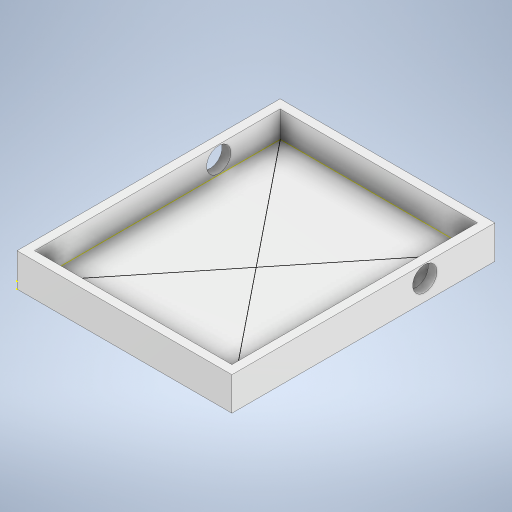
# Autodesk Inventor part: Case_3d_model2
Saved by Autodesk Inventor 2023 (Build 270158000, 158)
## iProperties
Created: 2023-03-21
Part Number: Case_3d_model2
Material: ABS Plastic
Document SubType Name: Sheet Metal
Designer: Inteli
Density: 1.06 g/cm^3
Sheet Metal Rule: Default
Appearance: Smooth - White
Author: Inteli
## iProperties of the stored document Case_3d_model_3DPrint.ipt
Created: 2023-03-23
Part Number: Case_3d_model_3DPrint
Material: Generic
Document SubType Name: Modeling
Designer: Inteli
Density: 1 g/cm^3
Appearance: Default
Author: Inteli
Autodesk Inventor part; units mm, degrees
ref_plane "YZ Plane" through (0, 0, 0) normal (1, 0, 0) x (0, 1, 0)
ref_plane "XZ Plane" through (0, 0, 0) normal (0, 1, 0) x (-1, 0, 0)
ref_plane "XY Plane" through (0, 0, 0) normal (0, 0, 1) x (1, 0, 0)
sketch "Sketch1" plane through (0, 0, 0) normal (0, 1, 0) x (-1, 0, 0)
  line L0 (0, 0) -> (0, -250)
  line L1 (-200, 0) -> (0, 0)
  line L2 (0, -250) -> (0, -300)
  line L3 (0, -300) -> (-200, -300)
  line L4 (-200, -300) -> (-230, -300)
  line L5 (-230, 0) -> (-200, 0)
  line L6 (-230, -300) -> (-245, -300)
  line L7 (-245, -300) -> (-245, 0)
  line L8 (-245, 0) -> (-230, 0)
  dimension "d0" = 250
  dimension "d4" = 50
  dimension "d12" = 30
  dimension "d24" = 15
  constraints: 18 end point, 2 horizontal, 2 perpendicular, 2 vertical
  measures "d0" distance of L0.start L0.end
  measures "d4" distance of L0.end L2.end
  measures "d12" distance of L3.end L4.end
  measures "d24" distance of L4.end L6.end
extrude "Extrusion1" add sketch "Sketch1" along normal blind 38
sketch "Sketch2" plane through (0, 38, 0) normal (0, 1, 0) x (1, 0, 0)
  line L0 (0, 300) -> (0, 0) projected
  line L1 (0, 0) -> (245, 0) projected
  line L2 (10, 10) -> (10, 290)
  line L3 (245, 300) -> (0, 300) projected
  line L4 (245, 0) -> (245, 300) projected
  line L5 (245, 290) -> (235, 290)
  line L6 (235, 290) -> (235, 10)
  line L7 (235, 290) -> (10, 290)
  line L8 (0, 300) -> (0, 0) projected
  line L9 (235, 10) -> (10, 10)
  dimension "d25" = 10
  constraints: 10 end point, 2 perpendicular, 1 point on line
  measures "d25" distance of L5.end L5.start
extrude "Extrusion2" cut sketch "Sketch2" against normal blind 30 contours L6 L9 L2 L7
sketch "Sketch5" plane through (0, 0, 0) normal (0, -1, 0) x (1, 0, 0)
  point P0 (0, 0)
sketch "Sketch6" plane through (0, 8, 0) normal (0, 1, 0) x (1, 0, 0)
  point P0 (0, 0)
sketch "Sketch7" plane through (0, 8, 0) normal (0, 1, 0) x (1, 0, 0)
  line L0 (10, 290) -> (235, 290) projected
  line L1 (235, 10) -> (10, 10) projected
  line L2 (235, 290) -> (10, 10)
  line L3 (10, 10) -> (10, 290) projected
  line L4 (235, 10) -> (10, 290)
  point P0 (0, 0)
  constraints: 4 end point
sketch "Sketch8" plane through (245, 0, 0) normal (1, 0, 0) x (0, 0, -1)
  line L0 (0, 38) -> (300, 38) projected
  line L1 (0, 0) -> (300, 0) projected
  line L2 (0, 0) -> (0, 38) projected
  line L3 (150, 38) -> (150, 8)
  line L4 (290, 8) -> (10, 8) projected
  line L5 (150, 8) -> (290, 8)
  line L6 (290, 38) -> (290, 8) projected
  line L7 (290, 8) -> (290, 38)
  line L8 (290, 38) -> (150, 38)
  line L9 (290, 38) -> (10, 38) projected
  line L10 (150, 8) -> (290, 38)
  line L11 (290, 38) -> (150, 38)
  line L12 (290, 8) -> (150, 38)
  circle A0 centre (220, 23) radius 13.9087
  constraints: 14 end point, 2 midpoint, 2 perpendicular, 1 centre point, 1 collinear, 1 horizontal, 1 vertical
extrude "Extrusion4" cut sketch "Sketch8" against normal blind 250 contours A0 L10 L12 | L12 L10 A0 | A0 L12 L10 | L10 L12 A0
equation "\"BendRadius\" = Thickness"
equation "\"BendReliefWidth\" = Thickness"
equation "\"BendReliefDepth\" = 0.5 * Thickness"
equation "\"CornerReliefSize\" = 4 * Thickness"
equation "\"MinimumRemnant\" = 2 * Thickness"
equation "\"TransitionRadius\" = BendRadius"
equation "\"JacobiRadiusSize\" = BendRadius"
equation "\"GapSize\" = Thickness"
equation "\"Thickness\" = 3.048"
body "Solid1"
